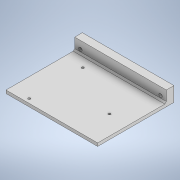
# Autodesk Inventor part: rig
Saved by Autodesk Inventor 2020.3 (Build 243373000, 373)
## iProperties
Created: 2020-07-10
Part Number: rig
Material: Generic
Document SubType Name: Modeling
Designer: OskarJohansson
Density: 1 g/cm^3
Appearance: Default
Author: OskarJohansson
## iProperties of the stored document _3DPrint.ipt
Created: 2020-07-10
Part Number: _3DPrint
Material: Generic
Document SubType Name: Modeling
Designer: OskarJohansson
Density: 1 g/cm^3
Appearance: Default
Author: OskarJohansson
Autodesk Inventor part; units mm, degrees
ref_plane "YZ Plane" through (0, 0, 0) normal (1, 0, 0) x (0, 1, 0)
ref_plane "XZ Plane" through (0, 0, 0) normal (0, 1, 0) x (-1, 0, 0)
ref_plane "XY Plane" through (0, 0, 0) normal (0, 0, 1) x (1, 0, 0)
sketch "Sketch1" plane through (0, 0, 0) normal (0, 1, 0) x (-1, 0, 0)
  line L0 (-60, 50) -> (60, 50)
  line L1 (60, 50) -> (60, -50)
  line L2 (60, -50) -> (-60, -50)
  line L3 (-60, -50) -> (-60, 50)
  line L4 (-60, 50) -> (60, -50) construction
  line L5 (60, 50) -> (-60, -50) construction
  point P0 (0, 0)
  dimension "d0" = 100
  dimension "d1" = 120
  constraints: 12 end point, 2 midpoint, 2 parallel, 1 horizontal, 1 perpendicular
  measures "d0" distance of L0.end L1.end
  measures "d1" distance of L1.end L2.end
extrude "Extrusion1" add sketch "Sketch1" along normal blind 5
sketch "Sketch2" plane through (0, 5, 0) normal (0, 1, 0) x (1, 0, 0)
  line L0 (-70.5402, 20) -> (79.21, 20) construction
  line L1 (-60, -50) -> (60, -50) projected
  line L2 (60, 50) -> (-60, 50)
  line L3 (-60, 50) -> (-60, 40)
  line L4 (-60, 40) -> (60, 40)
  line L5 (60, 40) -> (60, 50)
  line L6 (60, 50) -> (-60, 40) construction
  line L7 (-60, 50) -> (60, 40) construction
  line L8 (0, 70) -> (0, -70) projected
  line L9 (-60, 50) -> (-60, -50) projected
  line L10 (60, 50) -> (-60, 50) projected
  point P0 (0, 0)
  point P1 (0, 45)
  point P2 (0, 45)
  dimension "d4" = 70
  dimension "d5" = 10
  constraints: 14 end point, 3 midpoint, 2 collinear, 2 horizontal, 2 parallel, 1 perpendicular, 1 point on line
  measures "d4" distance between parallel lines of L1 L0
  measures "d5" distance of L2.end L3.end
extrude "Extrusion2" add sketch "Sketch2" along normal blind 15 contours L3 L2 L8 L4 | L8 L2 L5 L4
sketch "Sketch3" plane through (-60, 5, -40) normal (0, 0, 1) x (1, 0, 0)
  circle A0 centre (7.5, 5) radius 2.25
  line L0 (60, -9) -> (60, 19) construction
  circle A1 centre (112.5, 5) radius 2.25
  line L1 (120, 0) -> (0, 0) projected
  line L2 (0, -5) -> (120, -5) projected
  point P0 (60, -5)
  dimension "d8" = 4.5
  dimension "d9" = 105
  dimension "d22" = 10
  constraints: 2 centre point, 1 symmetric about line, 1 other
  measures "d8" diameter of A0
  measures "d9" distance of A1.centre A0.centre
  measures "d22" distance from line of L2 A1.centre
extrude "Extrusion3" cut sketch "Sketch3" against normal up to next
sketch "Sketch4" plane through (0, 5, 0) normal (0, 1, 0) x (1, 0, 0)
  circle A0 centre (-35, 25.4797) radius 1.5
  circle A1 centre (-35, -44.5203) radius 1.5
  circle A2 centre (35, -9.5203) radius 1.5
  line L0 (-101.4889, -9.5203) -> (42.7418, -9.5203) construction
  point P0 (0, 0)
  dimension "d13" = 70
  dimension "d14" = 70
  dimension "d15" = 3
  dimension "d16" = 35
  constraints: 3 centre point, 2 end point, 1 equal radius, 1 horizontal, 1 point on line, 1 other
  measures "d13" distance of A1.centre A0.centre
  measures "d14" horizontal distance of A2.centre A0.centre
  measures "d15" diameter of A2
  measures "d16" horizontal distance of point (0, 0) A0.centre
extrude "Extrusion4" cut sketch "Sketch4" against normal up to next
chamfer "Chamfer2" distance 2 angle 45 1 edges at (0, 5, -40)
chamfer "Chamfer3" distance 1 angle 45 4 edges at (-60, 0, 0) (0, 0, 50) (0, 0, -50) (60, 0, 0)
equation "\"d16\" = 0.5 * d14"
body "Solid1"
